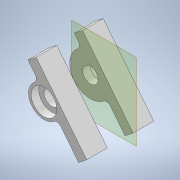
# Autodesk Inventor part: DUCT
Saved by Autodesk Inventor 2022 (Build 260153070, 153G)
## iProperties
Created: 2022-01-02
Part Number: DUCT
Material: Generic
Document SubType Name: Modeling
Designer: a laptop
Density: 1 g/cm^3
Appearance: Default
Author: a laptop
Autodesk Inventor part; units mm, degrees
ref_plane "YZ Plane" through (0, 0, 0) normal (1, 0, 0) x (0, 1, 0)
ref_plane "XZ Plane" through (0, 0, 0) normal (0, 1, 0) x (-1, 0, 0)
ref_plane "XY Plane" through (0, 0, 0) normal (0, 0, 1) x (1, 0, 0)
sketch "Sketch2" plane through (0, 0, 0) normal (0, 0, 1) x (1, 0, 0)
  circle A0 centre (-1.152, -1.2926) radius 1.5 projected
  line L0 (7.132, -6.8938) -> (-2.6673, 5.4354)
  arc A1 (-2.1291, 1.5439) -> (-3.0187, 1.056) centre (-1.152, -1.2926) ccw construction
  line L1 (7.132, -6.8938) -> (5.5664, -8.1383)
  line L2 (-4.233, 4.191) -> (-2.6673, 5.4354)
  line L3 (5.5664, -8.1383) -> (2.1197, -3.8018)
  line L4 (-2.1291, 1.5439) -> (-2.858, 2.461) construction
  arc A2 (-3.0187, 1.056) -> (-2.858, 2.461) centre (-3.6409, 1.8388) ccw
  arc A3 (2.1197, -3.8018) -> (0.7146, -3.6411) centre (1.3368, -4.424) ccw
  line L5 (-2.858, 2.461) -> (-4.233, 4.191)
  arc A4 (-3.0187, 1.056) -> (0.7146, -3.6411) centre (-1.152, -1.2926) ccw
  line L6 (2.1197, -3.8018) -> (1.3907, -2.8846) construction
  arc A5 (0.7146, -3.6411) -> (1.3907, -2.8846) centre (-1.152, -1.2926) ccw construction
  point P0 (0, 0)
  dimension "d0" = 1.5
  dimension "d1" = 2
  dimension "d3" = 90
  dimension "d4" = 90
  constraints: 14 end point, 11 point on circle, 6 tangent, 5 centre point, 5 perpendicular, 4 collinear, 1 concentric, 1 parallel, 2 other
  measures "d0" radial gap between concentric circles of A0 A1
  measures "d1" distance of L0.start L1.end
extrude "Extrusion1" add sketch "Sketch2" along normal blind 4
sketch "Sketch3" plane through (0, 0, 4) normal (0, 0, 1) x (1, 0, 0)
  circle A0 centre (-1.152, -1.2926) radius 2.5
  circle A1 centre (-1.152, -1.2926) radius 1.5 projected
  point P0 (0, 0)
  dimension "d7" = 5
  constraints: 1 centre point, 1 concentric
  measures "d7" diameter of A0
extrude "Extrusion2" cut sketch "Sketch3" against normal blind 1.5 contours A0 | A1
ref_plane "Work Plane1" through (0, 0, -5) normal (0, 0, -1) x (-1, 0, 0)
sketch "Sketch4" plane through (0, 0, -5) normal (0, 0, -1) x (-1, 0, 0)
  line L0 (-7.132, -6.8938) -> (2.6673, 5.4354) projected
  line L1 (-5.5664, -8.1383) -> (-7.132, -6.8938) projected
  line L2 (-2.1197, -3.8018) -> (-5.5664, -8.1383) projected
  arc A0 (-0.7146, -3.6411) -> (-2.1197, -3.8018) centre (-1.3368, -4.424) ccw projected
  arc A1 (2.858, 2.461) -> (3.0187, 1.056) centre (3.6409, 1.8388) ccw projected
  line L3 (4.233, 4.191) -> (2.858, 2.461) projected
  line L4 (2.6673, 5.4354) -> (4.233, 4.191) projected
  circle A2 centre (1.152, -1.2926) radius 1.5 projected
  arc A3 (-0.7146, -3.6411) -> (3.0187, 1.056) centre (1.152, -1.2926) ccw projected
  arc A4 (-1.3368, -4.424) -> (3.6409, 1.8388) centre (1.152, -1.2926) ccw
  line L5 (-2.1197, -3.8018) -> (-5.5664, -8.1383) projected
  arc A5 (-1.3368, -4.424) -> (-2.7419, -4.5846) centre (-1.959, -5.2068) ccw
  arc A6 (3.4802, 3.2439) -> (3.6409, 1.8388) centre (4.2631, 2.6217) ccw
  point P0 (0, 0)
  constraints: 6 centre point, 6 point on circle, 4 tangent, 2 point on line, 1 coincident, 1 concentric
extrude "Extrusion3" add sketch "Sketch4" along normal blind 4
sketch "Sketch5" plane through (0, 0, -9) normal (0, 0, -1) x (-1, 0, 0)
  line L0 (3.1278, 1.1933) -> (4.2928, -1.7607)
  line L1 (4.2928, -1.7607) -> (2.317, -4.2466)
  line L2 (2.317, -4.2466) -> (-0.8238, -3.7785)
  line L3 (-0.8238, -3.7785) -> (-1.9887, -0.8244)
  line L4 (-1.9887, -0.8244) -> (-0.0129, 1.6614)
  line L5 (-0.0129, 1.6614) -> (3.1278, 1.1933)
  line L6 (2.6673, 5.4354) -> (-7.132, -6.8938) projected
  circle A0 centre (1.152, -1.2926) radius 1.5 projected
  point P0 (0, 0)
  dimension "d13" = 5.5
  constraints: 12 end point, 1 coincident, 1 parallel, 13 other
  measures "d13" distance between parallel lines of L5 L2
extrude "Extrusion4" cut sketch "Sketch5" against normal blind 2.5
sketch "Sketch6" plane through (5.5664, -8.1383, 0) normal (-0.7828483, -0.6222126, 0) x (0, 0, 1)
  line L0 (-5, 0) -> (-5, 4.5394) projected
  line L1 (-5, 4) -> (0, 4)
  line L2 (0, 5.5394) -> (0, 0) projected
  line L3 (-5, 0) -> (-9, 0) projected
  line L4 (-5, 0) -> (0, 0)
  point P0 (0, 9.8345)
  dimension "d17" = 4
  constraints: 4 end point, 2 point on line, 1 collinear, 1 horizontal
  measures "d17" distance between parallel lines of L4 L1
extrude "Extrusion5" add sketch "Sketch6" against normal blind 2
sketch "Sketch7" plane through (0, 0, -9) normal (0, 0, -1) x (-1, 0, 0)
  line L0 (-5.5664, -8.1383) -> (-7.132, -6.8938) projected
  line L1 (-7.132, -6.8938) -> (-4.5773, -6.8938)
  line L2 (-5.5664, -8.1383) -> (-2.7419, -4.5846) projected
  point P0 (0, 0)
  constraints: 2 end point, 1 horizontal, 1 point on line
extrude "Extrusion6" cut sketch "Sketch7" against normal blind 14.7
body "Solid1"
